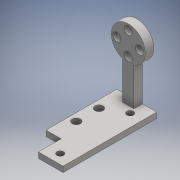
# Autodesk Inventor part: leverServoMount
Saved by Autodesk Inventor 2016 (Build 200138000, 138)
## iProperties
Created: 2016-05-02
Part Number: leverServoMount
Material: Generic
Document SubType Name: Modeling
Designer: mkepler
Density: 1 g/cm^3
Appearance: Default
Author: mkepler
Autodesk Inventor part; units mm, degrees
ref_plane "YZ Plane" through (0, 0, 0) normal (1, 0, 0) x (0, 1, 0)
ref_plane "XZ Plane" through (0, 0, 0) normal (0, 1, 0) x (-1, 0, 0)
ref_plane "XY Plane" through (0, 0, 0) normal (0, 0, 1) x (1, 0, 0)
sketch "Sketch1" plane through (0, 0, 0) normal (0, 1, 0) x (-1, 0, 0)
  arc A0 (3, -8.4853) -> (-3, -8.4853) centre (0, 0) ccw
  circle A1 centre (6, 0) radius 2.175
  circle A2 centre (0, -6) radius 2.175
  circle A3 centre (0, 6) radius 2.175
  circle A4 centre (-6, 0) radius 2.175
  line L0 (-3, -8.4853) -> (-3, -28.4853)
  line L1 (-3, -28.4853) -> (3, -28.4853)
  line L2 (3, -28.4853) -> (3, -8.4853)
  dimension "d0" = 18
  dimension "d1" = 4.35
  dimension "d2" = 6
  dimension "d3" = 4.35
  dimension "d4" = 6
  dimension "d5" = 4.35
  dimension "d6" = 6
  dimension "d7" = 4.35
  dimension "d8" = 6
  dimension "d13" = 6
  dimension "d66" = 20
  constraints: 6 end point, 5 centre point, 2 perpendicular, 2 point on circle, 1 coincident, 1 vertical
  measures "d0" diameter of A0
  measures "d1" diameter of A1
  measures "d2" distance of point (0, 0) A1.centre
  measures "d3" diameter of A2
  measures "d4" distance of point (0, 0) A2.centre
  measures "d5" diameter of A3
  measures "d6" distance of point (0, 0) A3.centre
  measures "d7" diameter of A4
  measures "d8" distance of point (0, 0) A4.centre
  measures "d13" distance of L0.end L1.end
  measures "d66" distance of L0.start L0.end
extrude "Extrusion1" add sketch "Sketch1" along normal blind 3
sketch "Sketch2" plane through (0, 3, 0) normal (0, 1, 0) x (1, 0, 0)
  line L0 (3, 28.4853) -> (-3, 28.4853) projected
  line L1 (-3, 28.4853) -> (3, 28.4853)
  line L2 (3, 28.4853) -> (3, 29.9853)
  line L3 (3, 29.9853) -> (-3, 29.9853)
  line L4 (-3, 29.9853) -> (-3, 28.4853)
  point P0 (0, 0)
  dimension "d14" = 6
  dimension "d15" = 1.5
  constraints: 8 end point, 2 parallel, 1 horizontal, 1 perpendicular
  measures "d14" distance of L3.end L2.end
  measures "d15" distance of L2.end L1.end
extrude "Extrusion2" add sketch "Sketch2" against normal blind 48
sketch "Sketch3" plane through (3, 3, -29.9853) normal (0, 0, -1) x (-1, 0, 0)
  line L0 (0, -3) -> (0, -48) projected
  line L1 (0, -48) -> (-3.5, -48)
  line L2 (-3.5, -48) -> (-3.5, 0)
  line L3 (-5.175, 0) -> (-0.825, 0) projected
  line L4 (-3.5, 0) -> (0, 0)
  line L5 (0, 0) -> (0, -48)
  line L6 (0, -48) -> (6, -48) projected
  line L7 (6.825, 0) -> (11.175, 0) projected
  line L8 (6, -48) -> (9.5, -48)
  line L9 (9.5, -48) -> (9.5, 0)
  line L10 (9.5, 0) -> (6, 0)
  line L11 (6, 0) -> (6, -48)
  line L12 (9.5, 0) -> (9.5, -48)
  line L13 (-3.5, -48) -> (-7.5, -48)
  line L14 (-7.5, -48) -> (-7.5, 0)
  line L15 (-7.5, 0) -> (-3.5, 0)
  line L16 (-3.5, 0) -> (-3.5, -48)
  line L17 (9.5, -48) -> (13.5, -48)
  line L18 (13.5, -48) -> (13.5, 0)
  line L19 (13.5, 0) -> (9.5, 0)
  line L20 (9.5, 0) -> (9.5, -48)
  point P0 (3, -3)
  dimension "d18" = 3.5
  dimension "d19" = 3.5
  dimension "d43" = 4
  dimension "d44" = 4
  constraints: 34 end point, 6 parallel, 5 horizontal, 5 perpendicular, 3 point on line
  measures "d18" distance of L0.end L1.end
  measures "d19" distance of L10.end L9.end
  measures "d43" distance of L14.end L15.end
  measures "d44" distance of L19.end L18.end
extrude "Extrusion3" add sketch "Sketch3" against normal blind 1.5
sketch "Sketch4" plane through (6.5, -45, -29.9853) normal (0, 0, -1) x (-1, 0, 0)
  circle A0 centre (2.5, 5) radius 1.75
  line L0 (-4, 0) -> (17, 0) projected
  line L1 (17, 0) -> (-4, 0) projected
  circle A1 centre (2.5, 42) radius 1.75
  line L2 (-2.5, 45) -> (15.5, 45) projected
  line L3 (-4, 48) -> (-4, 0) projected
  point P0 (6.5, 45)
  point P1 (0, 0)
  point P2 (21, 0)
  point P3 (0, 48)
  point P4 (3.5, 45)
  point P5 (9.5, 45)
  point P6 (9.5, 0)
  point P7 (3.5, 0)
  point P8 (13, 0)
  dimension "d23" = 3.5
  dimension "d26" = 3.5
  dimension "d28" = 3
  dimension "d45" = 6.5
  dimension "d46" = 6.5
  dimension "d78" = 37
  constraints: 2 centre point
  measures "d23" diameter of A0
  measures "d26" diameter of A1
  measures "d28" distance from line of A1.centre L2
  measures "d45" distance from line of L3 A1.centre
  measures "d46" distance from line of L3 A0.centre
  measures "d78" distance of A1.centre A0.centre
hole "Hole1" at (4, -40, -29.9853) at (4, -3, -29.9853) direction (0, 0, 1) diameter 3.5 depth 8 tip angle 118
sketch "Sketch5" plane through (6.5, -45, -29.9853) normal (0, 0, -1) x (-1, 0, 0)
  line L0 (0.0281, 45) -> (0.0281, 42)
  line L1 (0.0281, 42) -> (0.0281, 30)
  line L2 (0.0281, 30) -> (17, 30)
  line L3 (17, 48) -> (17, 0) projected
  circle A0 centre (13, 36) radius 2.175
  circle A1 centre (13, 24) radius 2.175
  dimension "d36" = 3
  dimension "d47" = 12
  dimension "d48" = 4.35
  dimension "d49" = 6
  dimension "d50" = 4
  dimension "d51" = 4.35
  dimension "d52" = 6
  dimension "d53" = 4
  constraints: 6 end point, 2 centre point, 1 perpendicular, 1 point on line, 1 vertical
  measures "d36" distance of L0.start L0.end
  measures "d47" distance of L0.end L1.end
  measures "d48" diameter of A0
  measures "d49" distance from line of L2 A0.centre
  measures "d50" distance from line of L3 A0.centre
  measures "d51" diameter of A1
  measures "d52" distance from line of A1.centre L2
  measures "d53" distance from line of L3 A1.centre
hole "Hole2" at (-6.5, -21, -29.9853) at (-6.5, -9, -29.9853) direction (0, 0, 1) diameter 4.35 depth 8 tip angle 118
sketch "Sketch6" plane through (10.5, -45, -29.9853) normal (0, 0, -1) x (-1, 0, 0)
  line L0 (0, 0) -> (13, 0)
  line L1 (21, 0) -> (0, 0) projected
  line L2 (13.5, 48) -> (21, 48) projected
  line L3 (13, 0) -> (13, 12)
  line L4 (12.675, 45) -> (12.675, 48) projected
  line L5 (17.25, 24) -> (29.25, 24) construction
  line L6 (21, 12) -> (17.25, 12)
  line L7 (21, 48) -> (21, 0) projected
  line L8 (21, 12) -> (21, 0)
  line L9 (21, 0) -> (13, 0)
  line L10 (13, 0) -> (13, 12)
  line L11 (13, 12) -> (21, 12)
  point P0 (10.5, 45)
  dimension "d61" = 13
  constraints: 16 end point, 2 collinear, 2 horizontal, 1 parallel, 1 perpendicular, 1 point on line
  measures "d61" distance of L0.start L0.end
extrude "Extrusion4" cut sketch "Sketch6" against normal through all
sketch "Sketch7" plane through (0, 3, 0) normal (0, 1, 0) x (1, 0, 0)
  line L0 (10.5, 29.9853) -> (-10.5, 29.9853) projected
  line L1 (-10.5, 29.9853) -> (-10.5, 28.4853) projected
  line L2 (-10.5, 29.9853) -> (-10.5, 28.4853)
  line L3 (-3, 28.4853) -> (-10.5, 28.4853) projected
  line L4 (-10.5, 28.4853) -> (-3, 28.4853)
  line L5 (-3, 8.4853) -> (-3, 28.4853) projected
  line L6 (-3, 28.4853) -> (-3, 8.4853)
  line L7 (10.5, 29.9853) -> (10.5, 28.4853) projected
  line L8 (-10.5, 29.9853) -> (10.5, 29.9853)
  line L9 (10.5, 29.9853) -> (10.5, 28.4853)
  line L10 (3, 28.4853) -> (3, 8.4853) projected
  line L11 (10.5, 28.4853) -> (3, 28.4853)
  line L12 (3, 28.4853) -> (3, 8.4853)
  arc A0 (-3, 8.4853) -> (3, 8.4853) centre (0, 0) ccw
  circle A1 centre (0, 6) radius 2.175
  circle A2 centre (-6.0102, 0) radius 2.175
  circle A3 centre (6, 0) radius 2.175
  circle A4 centre (0, -6) radius 2.175
  dimension "d67" = 4.35
  dimension "d68" = 6
  dimension "d69" = 4.35
  dimension "d70" = 6
  dimension "d71" = 4.35
  dimension "d72" = 6
  constraints: 14 end point, 5 centre point, 3 collinear, 2 perpendicular, 2 point on circle, 1 coincident, 1 horizontal, 1 vertical
  measures "d67" diameter of A1
  measures "d68" distance of point (0, 0) A1.centre
  measures "d69" diameter of A3
  measures "d70" distance of point (0, 0) A3.centre
  measures "d71" diameter of A4
  measures "d72" distance of point (0, 0) A4.centre
extrude "Extrusion5" add sketch "Sketch7" along normal blind 1.5
sketch "Sketch8" plane through (10.5, -45, -29.9853) normal (0, 0, -1) x (-1, 0, 0)
  line L0 (13, 0) -> (13, 12) projected
  line L1 (13, -0.1664) -> (13, 12)
  line L2 (13, 12) -> (21, 12) projected
  line L3 (13, 12) -> (21, 12)
  line L4 (0, 49.5) -> (21, 49.5) projected
  line L5 (21, 12) -> (21, 49.5)
  line L6 (21, 49.5) -> (0, 49.5)
  line L7 (0, 0) -> (13, 0) projected
  line L8 (0, 49.5) -> (0, 0)
  line L9 (0, 49.5) -> (0, 0) projected
  line L10 (0, 0) -> (13, 0)
  circle A0 centre (6.5, 42) radius 1.75 projected
  circle A1 centre (6.5, 42) radius 1.75
  circle A2 centre (17, 24) radius 2.175 projected
  circle A3 centre (17, 24) radius 2.175
  circle A4 centre (17, 36) radius 2.175 projected
  circle A5 centre (17, 36) radius 2.175
  circle A6 centre (6.5, 5) radius 1.75 projected
  circle A7 centre (6.5, 5) radius 1.75
  point P0 (10.5, 45)
  dimension "d75" = 3.5
  constraints: 12 end point, 4 centre point, 4 coincident, 4 perpendicular, 2 collinear
  measures "d75" diameter of A1
extrude "Extrusion6" add sketch "Sketch8" along normal blind 1.5
body "Solid1"
